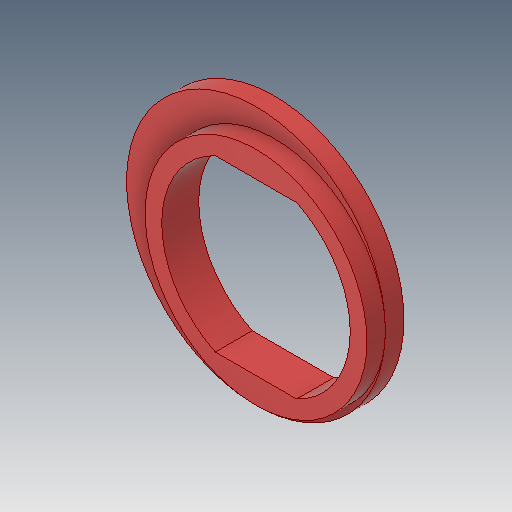
# Autodesk Inventor part: top_clip
Saved by Autodesk Inventor 2020.3 (Build 243373000, 373)
## iProperties
Created: 2021-02-25
Part Number: top_clip
Material: ABS Plastic
Document SubType Name: Modeling
Designer: paulg
Density: 1.06 g/cm^3
Appearance: Smooth - Red
Mass: 0.116115 g
Surface Area: 2.95554 cm^2
Volume: 0.109543 cm^3
Author: paulg
Autodesk Inventor part; units mm, degrees
ref_plane "YZ Plane" through (0, 0, 0) normal (1, 0, 0) x (0, 1, 0)
ref_plane "XZ Plane" through (0, 0, 0) normal (0, 1, 0) x (-1, 0, 0)
ref_plane "XY Plane" through (0, 0, 0) normal (0, 0, 1) x (1, 0, 0)
sketch "Sketch1" plane through (0, 0, 0) normal (0, 0, 1) x (1, 0, 0)
  line L0 (-2.2023, 4.6) -> (2.2023, 4.6)
  line L1 (-2.2023, -4.6) -> (2.2023, -4.6)
  line L2 (0, 0) -> (7.7204, 0) construction
  arc A0 (-2.2023, 4.6) -> (-2.2023, -4.6) centre (0, 0) ccw
  arc A1 (2.2023, -4.6) -> (2.2023, 4.6) centre (0, 0) ccw
  line L3 (0, 0) -> (-1, 0)
  circle A2 centre (-1, 0) radius 7
  line L4 (5.1, 0) -> (6, 0)
  dimension "d3" = 14
  dimension "d0" = 9.2
  dimension "d1" = 5.1
  dimension "d2" = 1
  dimension "d9" = 0.9
  constraints: 10 end point, 5 point on circle, 3 horizontal, 2 centre point, 2 coincident, 1 concentric, 1 horizontal alignment, 1 parallel, 1 point on line, 3 other
  measures "d0" distance between parallel lines of L1 L0
  measures "d1" radius of A0
  measures "d2" distance of L2.start L3.end
  measures "d9" distance of L4.end L4.start
extrude "Extrusion1" add sketch "Sketch1" along normal blind 1
sketch "Sketch2" plane through (-1, 0, 1) normal (0, 0, 1) x (1, 0, 0)
  arc A0 (3.2023, -4.6) -> (3.2023, 4.6) centre (1, 0) ccw projected
  line L0 (3.2023, -4.6) -> (-1.2023, -4.6) projected
  arc A1 (-1.2023, 4.6) -> (-1.2023, -4.6) centre (1, 0) ccw projected
  line L1 (-1.2023, 4.6) -> (3.2023, 4.6) projected
  circle A2 centre (0, 0) radius 7 projected
  circle A3 centre (1, 0) radius 6
  dimension "d6" = 12
  constraints: 1 centre point, 1 coincident
  measures "d6" diameter of A3
extrude "Extrusion2" add sketch "Sketch2" along normal blind 1 contours A3
body "Solid1"
